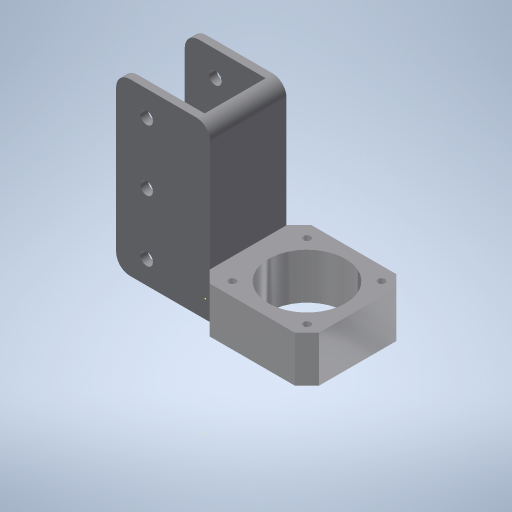
# Autodesk Inventor part: Nema 17 stepper motor.2ipt
Saved by Autodesk Inventor 2024 (Build 280153000, 153)
## iProperties
Created: 2012-11-28
Part Number: Nema 17 stepper motor.2ipt
Material: Generic
Document SubType Name: Modeling
Designer: Nico
Density: 1 g/cm^3
Appearance: Default
Author: Nico
Autodesk Inventor part; units mm, degrees
ref_plane "YZ Plane" through (0, 0, 0) normal (1, 0, 0) x (0, 1, 0)
ref_plane "XZ Plane" through (0, 0, 0) normal (0, 1, 0) x (-1, 0, 0)
ref_plane "XY Plane" through (0, 0, 0) normal (0, 0, 1) x (1, 0, 0)
sketch "Sketch1" plane through (0, 0, 0) normal (0, 0, 1) x (1, 0, 0)
  line L0 (0, 37.2) -> (5, 42.2)
  line L1 (37.2, 42.2) -> (42.2, 37.2)
  line L2 (42.2, 5) -> (37.2, 0)
  line L3 (5, 0) -> (0, 5)
  line L4 (0, 37.2) -> (0, 5)
  line L5 (37.2, 42.2) -> (5, 42.2)
  line L6 (42.2, 5) -> (42.2, 37.2)
  line L7 (5, 0) -> (37.2, 0)
  line L8 (0, 5) -> (0, 0)
  circle A0 centre (21.1, 21.1) radius 2.5
  circle A1 centre (5.6, 36.6) radius 1.5
  circle A2 centre (36.6, 36.6) radius 1.5
  circle A3 centre (36.6, 5.6) radius 1.5
  circle A4 centre (5.6, 5.6) radius 1.5
  dimension "d8" = 5
  dimension "d9" = 5
  dimension "d10" = 5
  dimension "d11" = 21.1
  dimension "d12" = 21.1
  dimension "d13" = 3
  dimension "d14" = 3
  dimension "d15" = 3
  dimension "d16" = 3
  dimension "d17" = 31
  dimension "d18" = 31
  dimension "d19" = 31
  dimension "d20" = 31
  dimension "d21" = 5.6
  dimension "d22" = 5.6
  dimension "d43" = 5.6
  dimension "d44" = 5.6
  dimension "d45" = 5.6
  dimension "d46" = 5.6
  dimension "d47" = 42.2
  constraints: 18 end point, 5 centre point, 4 parallel, 2 perpendicular, 1 horizontal
  measures "d8" distance of L8.end L3.start
  measures "d9" distance of L8.end L3.end
  measures "d10" diameter of A0
  measures "d11" distance from line of L4 A0.centre
  measures "d12" distance from line of L7 A0.centre
  measures "d13" diameter of A1
  measures "d14" diameter of A2
  measures "d15" diameter of A3
  measures "d16" diameter of A4
  measures "d17" distance of A3.centre A2.centre
  measures "d18" distance of A1.centre A2.centre
  measures "d19" distance of A4.centre A1.centre
  measures "d20" distance of A4.centre A3.centre
  measures "d21" distance from line of L5 A2.centre
  measures "d22" distance from line of L6 A2.centre
  measures "d43" distance from line of L5 A1.centre
  measures "d44" distance from line of L4 A1.centre
  measures "d45" distance from line of L4 A4.centre
  measures "d46" distance from line of L7 A3.centre
  measures "d47" distance between parallel lines of L7 L5
extrude "Extrusion1" add sketch "Sketch1" along normal blind 9.8
sketch "Sketch2" plane through (0, 0, 9.8) normal (0, 0, 1) x (1, 0, 0)
  circle A0 centre (21.1, 21.1) radius 2.5 projected
  circle A1 centre (5.6, 5.6) radius 1.5 projected
  circle A2 centre (36.6, 5.6) radius 1.5 projected
  circle A3 centre (36.6, 36.6) radius 1.5 projected
  circle A4 centre (5.6, 36.6) radius 1.5 projected
  line L0 (5, 42.2) -> (0, 37.2) projected
  line L1 (0, 37.2) -> (0, 5) projected
  line L2 (0, 5) -> (5, 0) projected
  line L3 (5, 0) -> (37.2, 0) projected
  line L4 (37.2, 0) -> (42.2, 5) projected
  line L5 (42.2, 5) -> (42.2, 37.2) projected
  line L6 (42.2, 37.2) -> (37.2, 42.2) projected
  line L7 (37.2, 42.2) -> (5, 42.2) projected
  point P0 (0, 0)
fillet "Fillet1" radius 0.25 8 edges at (21.1, 42.2, 9.8) (39.7, 39.7, 9.8) (42.2, 21.1, 9.8) (39.7, 2.5, 9.8) (21.1, 0, 9.8) (2.5, 2.5, 9.8) (0, 21.1, 9.8) (2.5, 39.7, 9.8)
extrude "Extrusion2" add sketch "Sketch2" along normal blind 31
sketch "Sketch3" plane through (0, 0, 40.8) normal (0, 0, 1) x (1, 0, 0)
  circle A0 centre (21.1, 21.1) radius 2.5 projected
  circle A1 centre (5.6, 36.6) radius 1.5 projected
  circle A2 centre (36.6, 36.6) radius 1.5 projected
  circle A3 centre (36.6, 5.6) radius 1.5 projected
  circle A4 centre (5.6, 5.6) radius 1.5 projected
  line L0 (5, 42.2) -> (0, 37.2) projected
  line L1 (0, 37.2) -> (0, 5) projected
  line L2 (0, 5) -> (5, 0) projected
  line L3 (5, 0) -> (37.2, 0) projected
  line L4 (37.2, 0) -> (42.2, 5) projected
  line L5 (42.2, 5) -> (42.2, 37.2) projected
  line L6 (42.2, 37.2) -> (37.2, 42.2) projected
  line L7 (37.2, 42.2) -> (5, 42.2) projected
  point P0 (0, 0)
fillet "Fillet2" radius 0.25 8 edges at (21.1, 42.2, 40.8) (39.7, 39.7, 40.8) (42.2, 21.1, 40.8) (39.7, 2.5, 40.8) (21.1, 0, 40.8) (2.5, 2.5, 40.8) (0, 21.1, 40.8) (2.5, 39.7, 40.8)
extrude "Extrusion3" add sketch "Sketch3" along normal blind 7.75
sketch "Sketch4" plane through (0, 0, 48.55) normal (0, 0, 1) x (1, 0, 0)
  circle A0 centre (21.1, 21.1) radius 2.5 projected
  circle A1 centre (21.1, 21.1) radius 16
  point P0 (0, 0)
  dimension "d31" = 32
  constraints: 1 centre point, 1 coincident
  measures "d31" diameter of A1
extrude "Extrusion4" cut sketch "Sketch4" against normal blind 0.6
sketch "Sketch5" plane through (21.1, 21.1, 47.95) normal (0, 0, 1) x (1, 0, 0)
  circle A0 centre (0, 0) radius 2.5 projected
  circle A1 centre (0, 0) radius 16 projected
  circle A2 centre (0, 0) radius 11
  point P0 (-21.1, -21.1)
  dimension "d35" = 22
  constraints: 1 centre point, 1 coincident
  measures "d35" diameter of A2
extrude "Extrusion5" add sketch "Sketch5" along normal blind 2.2 contours A2
fillet "Fillet3" radius 0.5 1 edges at (10.1, 21.1, 50.15)
sketch "Sketch6" plane through (21.1, 21.1, 50.15) normal (0, 0, 1) x (1, 0, 0)
  circle A0 centre (0, 0) radius 2.5 projected
  point P0 (-21.1, -21.1)
extrude "Extrusion6" add sketch "Sketch6" along normal blind 22.5
fillet "Fillet4" radius 0.5 1 edges at (18.6, 21.1, 72.65)
sketch "Sketch7" plane through (0, 0, 48.55) normal (0, 0, 1) x (1, 0, 0)
  circle A0 centre (21.1, 21.1) radius 16 projected
  circle A1 centre (5.6, 5.6) radius 1.5 projected
  circle A2 centre (36.6, 5.6) radius 1.5 projected
  circle A3 centre (36.6, 36.6) radius 1.5 projected
  circle A4 centre (5.6, 36.6) radius 1.5 projected
  line L0 (5, 42.2) -> (0, 37.2) projected
  line L1 (0, 37.2) -> (0, 5) projected
  line L2 (0, 5) -> (5, 0) projected
  line L3 (5, 0) -> (37.2, 0) projected
  line L4 (37.2, 0) -> (42.2, 5) projected
  line L5 (42.2, 5) -> (42.2, 37.2) projected
  line L6 (42.2, 37.2) -> (37.2, 42.2) projected
  line L7 (37.2, 42.2) -> (5, 42.2) projected
  point P0 (0, 0)
extrude "Extrusion7" add sketch "Sketch7" along normal blind 6.35
sketch "Sketch8" plane through (5, 0, 40.8) normal (0, -1, 0) x (1, 0, 0)
  point P0 (-5, -40.8)
sketch "Sketch9" plane through (5, 0, 40.8) normal (0, -1, 0) x (1, 0, 0)
  line L0 (0, 14.1) -> (-5, 14.1) projected
  line L1 (37.2, 0) -> (37.2, 14.1) projected
  line L2 (-5, 14.1) -> (37.2, 14.1)
  line L3 (37.2, 14.1) -> (37.2, 7.75)
  line L4 (37.2, 7.75) -> (-5, 7.75)
  line L5 (-5, 7.75) -> (-5, 14.1)
  line L6 (-5, 7.75) -> (48.466, 7.75)
  line L7 (48.466, 7.75) -> (48.466, -59.7117)
  line L8 (48.466, -59.7117) -> (-5, -59.7117)
  line L9 (-5, -59.7117) -> (-5, 7.75)
  point P0 (-5, -40.8)
  dimension "d50" = 6.35
  constraints: 16 end point, 4 parallel, 2 horizontal, 2 perpendicular, 1 point on line
  measures "d50" distance between parallel lines of L2 L4
extrude "Extrusion8" cut sketch "Sketch9" against normal blind 98.4 contours L4 L6 L7 L8 L9
sketch "Sketch10" plane through (21.1, 21.1, 48.55) normal (0, 0, -1) x (-1, 0, 0)
  circle A0 centre (0, 0) radius 11 projected
  circle A1 centre (0, 0) radius 2.5 projected
  circle A2 centre (0, 0) radius 2.5 projected
  point P0 (21.1, -21.1)
extrude "Extrusion9" cut sketch "Sketch10" against normal blind 76.85 contours A0 | A1
sketch "Sketch11" plane through (0, 5, 54.9) normal (-1, 0, 0) x (0, 0, 1)
  line L0 (-6.35, -5) -> (-6.35, 0) projected
  line L1 (0, 37.2) -> (-6.35, 37.2)
  line L2 (-6.35, 37.2) -> (-6.35, -5)
  line L3 (-6.35, -5) -> (0, -5)
  line L4 (0, -5) -> (0, 37.2)
  point P0 (-54.9, -5)
  constraints: 8 end point, 2 parallel, 1 horizontal, 1 perpendicular
extrude "Extrusion10" add sketch "Sketch11" along normal blind 16.9926
sketch "Sketch12" plane through (0, 5, 54.9) normal (1, 0, 0) x (0, 0, -1)
  line L0 (6.35, 32.2) -> (0, 32.2) projected
  line L1 (6.35, 37.2) -> (6.35, 32.2) projected
  line L2 (0, 37.2) -> (6.35, 37.2) projected
  line L3 (0, 32.2) -> (0, 37.2) projected
  line L4 (6.35, 0) -> (0, 0) projected
  line L5 (0, -5) -> (0, 0) projected
  line L6 (6.35, -5) -> (0, -5) projected
  line L7 (6.35, 0) -> (6.35, -5) projected
  point P0 (54.9, -5)
extrude "Extrusion11" add sketch "Sketch12" along normal blind 3.9926
sketch "Sketch13" plane through (3.9926, 5, 54.9) normal (1, 0, 0) x (0, 0, -1)
  line L0 (6.35, 36.1926) -> (0, 36.1926) projected
  line L1 (6.35, 36.1926) -> (6.35, 37.2) projected
  line L2 (6.35, 37.2) -> (0, 37.2) projected
  line L3 (0, 37.2) -> (0, 36.1926) projected
  line L4 (0, -3.9926) -> (6.35, -3.9926) projected
  line L5 (0, -3.9926) -> (0, -5) projected
  line L6 (0, -5) -> (6.35, -5) projected
  line L7 (6.35, -5) -> (6.35, -3.9926) projected
  point P0 (54.9, -5)
extrude "Extrusion12" add sketch "Sketch13" along normal blind 3.9926
sketch "Sketch14" plane through (-16.9926, 5, 54.9) normal (-1, 0, 0) x (0, 0, 1)
  line L0 (0, -5) -> (0, 0) projected
  line L1 (-6.35, 0) -> (-6.35, 32.2) projected
  line L2 (0, -5) -> (-6.35, -5)
  line L3 (-6.35, -5) -> (-6.35, 3.4074)
  line L4 (-6.35, 3.4074) -> (0, 3.4074)
  line L5 (0, 3.4074) -> (0, -5)
  line L6 (-6.35, 37.2) -> (0, 37.2) projected
  line L7 (0, 37.2) -> (-6.35, 37.2)
  line L8 (-6.35, 37.2) -> (-6.35, 28.7926)
  line L9 (-6.35, 28.7926) -> (0, 28.7926)
  line L10 (0, 28.7926) -> (0, 37.2)
  point P0 (-54.9, -5)
  point P1 (-3.175, 28.7926)
  dimension "d61" = 8.4074
  dimension "d62" = 8.4074
  constraints: 16 end point, 4 parallel, 2 horizontal, 2 perpendicular, 2 point on line, 1 midpoint
  measures "d61" distance between parallel lines of L2 L4
  measures "d62" distance from line of point (-3.175, 28.793) L6
extrude "Extrusion13" add sketch "Sketch14" along normal blind 25.4
sketch "Sketch15" plane through (-42.3926, 5, 54.9) normal (-1, 0, 0) x (0, 0, 1)
  line L0 (0, 3.4074) -> (-6.35, 3.4074)
  line L1 (-6.35, 3.4074) -> (-6.35, 0.2324)
  line L2 (-6.35, 0.2324) -> (0, 0.2324)
  line L3 (0, 0.2324) -> (0, 3.4074)
  line L4 (0, 37.2) -> (-6.35, 37.2) projected
  line L5 (-6.35, 37.2) -> (0, 37.2) construction
  line L6 (0, 37.2) -> (-6.35, 37.2) projected
  line L7 (-6.35, 37.2) -> (0, 37.2) projected
  line L8 (0, -5) -> (0, 3.4074) projected
  line L9 (0, 3.4074) -> (-6.35, 3.4074) projected
  line L10 (-6.35, 3.4074) -> (-6.35, -5) projected
  line L11 (-6.35, -5) -> (0, -5) projected
  line L12 (0, 28.7926) -> (0, 37.2) projected
  line L13 (-6.35, 37.2) -> (-6.35, 28.7926) projected
  line L14 (0, 28.7926) -> (-6.35, 28.7926)
  line L15 (-6.35, 28.7926) -> (-6.35, 31.9676)
  line L16 (-6.35, 31.9676) -> (0, 31.9676)
  line L17 (0, 31.9676) -> (0, 28.7926)
  line L18 (0, 37.2) -> (-6.35, 37.2) projected
  line L19 (-6.35, 37.2) -> (-6.35, 28.7926) projected
  line L20 (-6.35, 28.7926) -> (0, 28.7926) projected
  line L21 (0, 28.7926) -> (0, 37.2) projected
  point P0 (-54.9, -5)
  point P1 (0, 31.9676)
  point P2 (0, 0.2324)
  point P3 (-6.35, 0.2324)
  dimension "d66" = 3.175
  dimension "d68" = 3.175
  constraints: 16 end point, 4 parallel, 2 horizontal, 2 perpendicular, 1 point on line
  measures "d66" distance between parallel lines of L2 L0
  measures "d68" distance between parallel lines of L14 L16
extrude "Extrusion14" cut sketch "Sketch15" against normal blind 39.1 contours L8 L11 L10 L2 | L12 L16 L13 L4
chamfer "Chamfer1" distance 5 angle 45 2 edges at (-3.2926, 0, 51.725) (-3.2926, 42.2, 51.725)
sketch "Sketch16" plane through (42.2, 5, 48.55) normal (0, 0, -1) x (-1, 0, 0)
  point P0 (42.2, -5)
sketch "Sketch17" plane through (0, 0, 54.9) normal (0, 0, 1) x (1, 0, 0)
  line L0 (-3.2926, 36.9676) -> (-42.3926, 36.9676) projected
  line L1 (-42.3926, 5.2324) -> (-3.2926, 5.2324) projected
  line L2 (-3.2926, 36.9676) -> (-16.9772, 36.9676)
  line L3 (-16.9772, 36.9676) -> (-16.9772, 5.2324)
  line L4 (-16.9772, 5.2324) -> (-3.2926, 5.2324)
  line L5 (-3.2926, 5.2324) -> (-3.2926, 36.9676)
  point P0 (0, 0)
  constraints: 8 end point, 2 parallel, 1 horizontal, 1 perpendicular, 1 point on line
extrude "Extrusion15" add sketch "Sketch17" along normal blind 39.1
sketch "Sketch18" plane through (42.2, 5, 48.55) normal (0, 0, -1) x (-1, 0, 0)
  line L0 (59.1926, 3.4074) -> (59.1926, 28.7926) projected
  line L1 (84.5926, 0.2324) -> (84.5926, 3.4074) projected
  line L2 (59.1926, 3.4074) -> (84.5926, 3.4074)
  line L3 (84.5926, 3.4074) -> (84.5926, 0.2324)
  line L4 (84.5926, 0.2324) -> (59.1926, 0.2324)
  line L5 (59.1926, 0.2324) -> (59.1926, 3.4074)
  line L6 (59.1926, 28.7926) -> (84.5926, 28.7926) projected
  line L7 (59.1926, 32.131) -> (84.5926, 32.131)
  line L8 (84.5926, 32.131) -> (84.5926, 28.7926)
  line L9 (84.5926, 28.7926) -> (59.1926, 28.7926)
  line L10 (59.1926, 28.7926) -> (59.1926, 32.131)
  point P0 (42.2, -5)
  constraints: 16 end point, 4 parallel, 2 horizontal, 2 perpendicular, 1 point on line
extrude "Extrusion16" add sketch "Sketch18" along normal blind 12.7
sketch "Sketch19" plane through (42.2, 5, 48.55) normal (0, 0, 1) x (1, 0, 0)
  line L0 (-84.5926, 31.9676) -> (-57.74, 31.9676)
  line L1 (-57.74, 31.9676) -> (-57.74, 35.8031)
  line L2 (-57.74, 35.8031) -> (-84.5926, 35.8031)
  line L3 (-84.5926, 35.8031) -> (-84.5926, 31.9676)
  point P0 (-42.2, -5)
  constraints: 8 end point, 2 parallel, 1 horizontal, 1 perpendicular
extrude "Extrusion17" cut sketch "Sketch19" against normal blind 25.8
sketch "Sketch20" plane through (0, 0, 94) normal (0, 0, 1) x (1, 0, 0)
  line L0 (-3.2926, 36.9676) -> (-16.9772, 36.9676) projected
  line L1 (-16.9772, 36.9676) -> (-16.9772, 5.2324) projected
  line L2 (-16.9772, 5.2324) -> (-3.2926, 5.2324) projected
  line L3 (-3.2926, 5.2324) -> (-3.2926, 36.9676) projected
  point P0 (0, 0)
extrude "Extrusion18" add sketch "Sketch20" along normal blind 12.7
sketch "Sketch21" plane through (0, 0, 54.9) normal (0, 0, 1) x (1, 0, 0)
  line L0 (-16.9772, 5.2324) -> (-16.9772, 36.9676) projected
  line L1 (-16.9772, 36.9676) -> (-42.3926, 36.9676) projected
  line L2 (-42.3926, 33.7926) -> (-42.3926, 36.9676) projected
  line L3 (-16.9926, 33.7926) -> (-42.3926, 33.7926) projected
  line L4 (-16.9926, 8.4074) -> (-16.9926, 33.7926) projected
  line L5 (-16.9926, 8.4074) -> (-42.3926, 8.4074) projected
  line L6 (-42.3926, 5.2324) -> (-42.3926, 8.4074) projected
  line L7 (-42.3926, 5.2324) -> (-16.9772, 5.2324) projected
  point P0 (0, 0)
extrude "Extrusion19" add sketch "Sketch21" along normal blind 51.95
sketch "Sketch22" plane through (-16.9772, 5.2324, 106.7) normal (1, 0, 0) x (0, 0, -1)
  line L0 (0, 0) -> (-13.0158, 0)
  line L1 (-13.0158, 0) -> (-13.0158, 37.0534)
  line L2 (-13.0158, 37.0534) -> (0, 37.0534)
  line L3 (0, 37.0534) -> (0, 0)
  point P0 (106.7, -5.2324)
  constraints: 8 end point, 2 parallel, 1 horizontal, 1 perpendicular
extrude "Extrusion20" cut sketch "Sketch22" against normal blind 71.05
sketch "Sketch23" plane through (-3.2926, 5.2324, 48.55) normal (0, -1, 0) x (1, 0, 0)
  line L0 (-13.7, -12.7) -> (-39.1, -12.7) projected
  line L1 (-26.4, -12.7) -> (-26.4, 58.15)
  line L2 (0, 58.15) -> (-39.1, 58.15) projected
  line L3 (-26.4, 58.15) -> (-26.4, 47.7614)
  circle A0 centre (-26.4, 47.7614) radius 2.6289
  line L4 (-26.4, 47.7614) -> (-26.4, 22.3614)
  line L5 (-26.4, 22.3614) -> (-26.4, -3.0386)
  circle A1 centre (-26.4, 22.3614) radius 2.6289
  circle A2 centre (-26.4, -3.0386) radius 2.6289
  point P0 (3.2926, -48.55)
  dimension "d86" = 10.3886
  dimension "d87" = 5.2578
  dimension "d88" = 25.4
  dimension "d89" = 25.4
  dimension "d90" = 5.2578
  dimension "d91" = 5.2578
  constraints: 8 end point, 4 point on line, 3 centre point, 3 coincident, 1 midpoint, 1 vertical
  measures "d86" distance of L1.end L3.end
  measures "d87" diameter of A0
  measures "d88" distance of L4.start L4.end
  measures "d89" distance of L4.end L5.end
  measures "d90" diameter of A1
  measures "d91" diameter of A2
extrude "Extrusion21" cut sketch "Sketch23" against normal blind 133.45
sketch "Sketch24" plane through (0, 0, 106.7) normal (0, 0, 1) x (1, 0, 0)
  line L0 (-3.2926, 5.2324) -> (-42.3926, 5.2324) projected
  line L1 (-3.2926, 36.9676) -> (-9.6426, 36.9676)
  line L2 (-9.6426, 36.9676) -> (-9.6426, 5.2324)
  line L3 (-9.6426, 5.2324) -> (-3.2926, 5.2324)
  line L4 (-3.2926, 5.2324) -> (-3.2926, 36.9676)
  point P0 (0, 0)
  dimension "d95" = 6.35
  constraints: 8 end point, 2 parallel, 1 horizontal, 1 perpendicular, 1 point on line
  measures "d95" distance between parallel lines of L2 L4
extrude "Extrusion22" add sketch "Sketch24" along normal blind 6.35
sketch "Sketch25" plane through (-3.2926, 5.2324, 48.55) normal (0, -1, 0) x (1, 0, 0)
  line L0 (-6.35, 58.15) -> (-6.35, 64.5) projected
  line L1 (-6.35, 58.15) -> (52.4716, 58.15)
  line L2 (52.4716, 58.15) -> (52.4716, 64.5)
  line L3 (52.4716, 64.5) -> (-6.35, 64.5)
  line L4 (-6.35, 64.5) -> (-6.35, 58.15)
  point P0 (3.2926, -48.55)
  constraints: 8 end point, 2 parallel, 1 horizontal, 1 perpendicular
extrude "Extrusion23" add sketch "Sketch25" along normal blind 7.6
sketch "Sketch26" plane through (-3.2926, 5.2324, 48.55) normal (0, 1, 0) x (1, 0, 0)
  line L0 (0, -58.15) -> (0, -64.5) projected
  line L1 (52.4716, -64.5) -> (0, -64.5) projected
  line L2 (52.4716, -58.15) -> (52.4716, -64.5) projected
  line L3 (0, -58.15) -> (52.4716, -58.15) projected
  point P0 (3.2926, 48.55)
extrude "Extrusion24" add sketch "Sketch26" along normal blind 55.35
sketch "Sketch27" plane through (0, 0, 54.9) normal (0, 0, 1) x (1, 0, 0)
  line L0 (-3.2926, 36.9676) -> (-3.2926, 5.2324) projected
  line L1 (-3.2926, 5.2324) -> (-3.2926, 5) projected
  line L2 (1.7074, 0) -> (-3.2926, 5) projected
  line L3 (37.2, 0) -> (1.7074, 0) projected
  line L4 (37.2, 0) -> (42.2, 5) projected
  line L5 (42.2, 5) -> (42.2, 37.2) projected
  line L6 (42.2, 37.2) -> (37.2, 42.2) projected
  line L7 (37.2, 42.2) -> (1.7074, 42.2) projected
  line L8 (-3.2926, 37.2) -> (1.7074, 42.2) projected
  line L9 (-3.2926, 37.2) -> (-3.2926, 36.9676) projected
  circle A0 centre (5.6, 36.6) radius 1.5 projected
  circle A1 centre (36.6, 36.6) radius 1.5 projected
  circle A2 centre (36.6, 5.6) radius 1.5 projected
  circle A3 centre (5.6, 5.6) radius 1.5 projected
  circle A4 centre (21.1, 21.1) radius 16 projected
  line L10 (-3.2926, -11.2491) -> (64.8812, -11.2491)
  line L11 (64.8812, -11.2491) -> (64.8812, 73.1738)
  line L12 (64.8812, 73.1738) -> (-3.2926, 73.1738)
  line L13 (-3.2926, 73.1738) -> (-3.2926, -11.2491)
  point P0 (0, 0)
  constraints: 8 end point, 2 parallel, 1 horizontal, 1 perpendicular
extrude "Extrusion25" cut sketch "Sketch27" along normal blind 194.15 contours L13 L12 L11 L10 L2 L3 L4 L5 L6 L7 L8 | A0 | A1 | A2 | A3
sketch "Sketch28" plane through (-3.2926, -2.3676, 113.05) normal (1, 0, 0) x (0, 0, -1)
  line L0 (6.35, 10.775) -> (6.35, 36.1602) projected
  line L1 (0, 0) -> (0, 7.3676) projected
  line L2 (6.35, 0) -> (0, 0) projected
  line L3 (6.35, 7.3676) -> (6.35, 0) projected
  line L4 (6.35, 7.3676) -> (0, 7.3676) projected
  point P0 (113.05, 2.3676)
extrude "Extrusion26" cut sketch "Sketch28" against normal blind 28.6
sketch "Sketch29" plane through (42.2, 5, 113.05) normal (1, 0, 0) x (0, 0, -1)
  line L0 (6.35, 0) -> (0, 0) projected
  line L1 (6.35, 0) -> (-3.466, 0)
  line L2 (-3.466, 0) -> (-3.466, 41.9331)
  line L3 (-3.466, 41.9331) -> (6.35, 41.9331)
  line L4 (6.35, 41.9331) -> (6.35, 0)
  line L5 (6.35, 0) -> (-14.0561, 0)
  line L6 (-14.0561, 0) -> (-14.0561, -9.0915)
  line L7 (-14.0561, -9.0915) -> (6.35, -9.0915)
  line L8 (6.35, -9.0915) -> (6.35, 0)
  point P0 (113.05, -5)
  point P1 (1.8156, 0)
  constraints: 16 end point, 4 parallel, 2 horizontal, 2 perpendicular
extrude "Extrusion27" cut sketch "Sketch29" against normal blind 115.4
sketch "Sketch30" plane through (42.2, 5, 48.55) normal (0, 0, -1) x (-1, 0, 0)
  line L0 (59.1926, 31.9676) -> (45.4926, 31.9676) projected
  line L1 (45.4926, 31.9676) -> (45.4926, 32.2) projected
  line L2 (40.4926, 37.2) -> (45.4926, 32.2) projected
  line L3 (40.4926, 37.2) -> (5, 37.2) projected
  line L4 (0, 32.2) -> (5, 37.2) projected
  line L5 (0, 0) -> (0, 32.2) projected
  line L6 (5, -5) -> (0, 0) projected
  line L7 (5, -5) -> (40.4926, -5) projected
  line L8 (45.4926, 0) -> (40.4926, -5) projected
  line L9 (45.4926, 0) -> (45.4926, 0.2324) projected
  line L10 (45.4926, 0.2324) -> (59.1926, 0.2324) projected
  line L11 (59.1926, 28.7926) -> (59.1926, 3.4074) projected
  circle A0 centre (21.1, 16.1) radius 16 projected
  circle A1 centre (36.6, 0.6) radius 1.5 projected
  circle A2 centre (5.6, 0.6) radius 1.5 projected
  circle A3 centre (5.6, 31.6) radius 1.5 projected
  circle A4 centre (36.6, 31.6) radius 1.5 projected
  line L12 (59.1926, 28.7926) -> (59.1926, 31.9676) projected
  line L13 (59.1926, 0.2324) -> (59.1926, 3.4074) projected
  point P0 (42.2, -5)
extrude "Extrusion28" add sketch "Sketch30" along normal up to surface (12.7 mm away)
chamfer "Chamfer2" distance 8.25 angle 45 1 edges at (-16.9926, 21.1, 35.85)
chamfer "Chamfer3" distance 8.25 angle 45 1 edges at (-16.9926, 21.1, 106.7)
fillet "Fillet7" radius 5.75 5 edges at (-3.2926, 21.1, 106.7) (-42.3926, 35.3801, 106.7) (-42.3926, 6.8199, 106.7) (-42.3926, 6.8199, 35.85) (-42.3926, 35.3801, 35.85)
body "Solid1"
